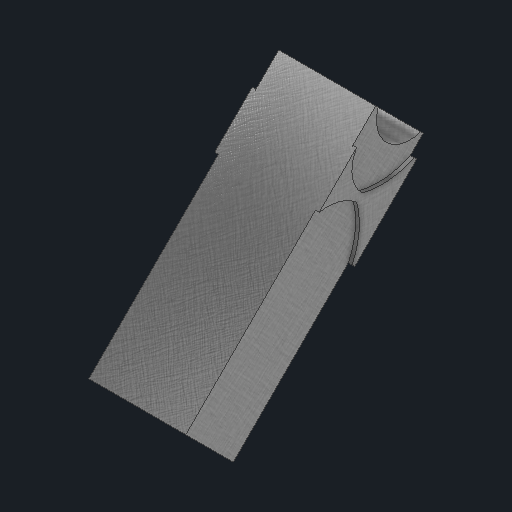
# Autodesk Inventor part: McCrea_paza_Walle
Saved by Autodesk Inventor 2022 (Build 260153000, 153)
## iProperties
Created: 2022-01-25
Part Number: McCrea_paza_Walle
Material: Generic
Document SubType Name: Modeling
Designer: Lukas
Density: 1 g/cm^3
Appearance: Honed - Dark Gray
Author: Lukas
Autodesk Inventor part; units mm, degrees
ref_plane "YZ Plane" through (0, 0, 0) normal (1, 0, 0) x (0, 1, 0)
ref_plane "XZ Plane" through (0, 0, 0) normal (0, 1, 0) x (-1, 0, 0)
ref_plane "XY Plane" through (0, 0, 0) normal (0, 0, 1) x (1, 0, 0)
sketch "Sketch1" plane through (0, 0, 0) normal (1, 0, 0) x (0, 1, 0)
  line L0 (0, 0) -> (6.364, 6.364)
  line L1 (0, 0) -> (10.533, 0) construction
  line L2 (0, 0) -> (36, 0) construction
  line L3 (-19.0919, 31.8198) -> (-25.4558, 25.4558)
  line L4 (-19.0919, 31.8198) -> (6.364, 6.364)
  line L5 (-25.4558, 25.4558) -> (0, 0)
  dimension "d0" = 9
  dimension "d1" = 45
  dimension "d2" = 36
  dimension "d15" = 9
  constraints: 12 end point, 2 horizontal, 1 parallel, 1 perpendicular, 1 point on line
  measures "d0" distance of L0.start L0.end
  measures "d1" angle of L1 L0
  measures "d2" distance of L0.start L3.end
  measures "d15" distance of L3.start L3.end
extrude "Extrusion4" add sketch "Sketch1" along normal blind 13
sketch "Sketch4" plane through (13, 0, 0) normal (1, 0, 0) x (0, 0, -1)
  line L0 (0, 0) -> (-6.364, 6.364) projected
  line L1 (-3.182, 3.182) -> (-1.7678, 1.7678)
  line L2 (-3.182, 3.182) -> (-1.7678, 4.5962)
  circle A0 centre (-1.7678, 4.5962) radius 4.5
  point P0 (-6.0324, 6.0324)
  point P1 (-0.3315, 0.3315)
  dimension "d18" = 2
  dimension "d19" = 2
  dimension "d20" = 9
  constraints: 4 end point, 1 centre point, 1 coincident, 1 midpoint, 1 perpendicular, 1 point on line
  measures "d18" distance of L1.start L1.end
  measures "d19" distance of L1.start L2.end
  measures "d20" diameter of A0
extrude "Extrusion5" cut sketch "Sketch4" against normal blind 13 contours L0 A0 picked at (-2.8444, 1.8095)
sketch "Sketch8" plane through (13, 0, 0) normal (0, -0.7071068, -0.7071068) x (-1, 0, 0)
  line L0 (0, -36) -> (0, 0) projected
  line L1 (0, -1.9255) -> (0, -2.4255)
  line L2 (0, -2.4255) -> (-0.5, -2.4255)
  line L3 (13, -36) -> (13, 0) projected
  line L4 (13, -13.6899) -> (13, -14.1899)
  line L5 (13, -14.1899) -> (13.5, -14.1899)
  line L6 (13.5, -14.1899) -> (-0.5, -14.1899)
  line L7 (-0.5, -14.1899) -> (-0.5, -2.4255)
  line L8 (-0.5, -2.4255) -> (13.5, -2.4255)
  line L9 (13.5, -2.4255) -> (13.5, -14.1899)
  dimension "d31" = 0.5
  dimension "d32" = 0.5
  dimension "d33" = 0.5
  dimension "d34" = 0.5
  constraints: 16 end point, 4 point on line, 2 horizontal, 2 parallel, 2 perpendicular
  measures "d31" distance of L1.start L1.end
  measures "d32" distance of L1.end L2.end
  measures "d33" distance of L4.start L4.end
  measures "d34" distance of L4.end L5.end
extrude "Extrusion7" add sketch "Sketch8" along normal blind 0.5
sketch "Sketch9" plane through (13, 0, 0) normal (1, 0, 0) x (0, 0, -1)
  line L0 (-1.7151, -1.7151) -> (-10.0338, -10.0338) projected
  line L1 (-5.8744, -5.8744) -> (-12.2384, 0.4895)
  line L2 (-6.364, 6.364) -> (-31.8198, -19.0919) projected
  line L3 (-9.0564, -2.6925) -> (-8.7029, -2.3389)
  line L4 (-9.0564, -2.6925) -> (-9.41, -3.046)
  line L5 (-1.7151, -1.7151) -> (0, 0) projected
  arc A0 (-8.7029, -2.3389) -> (-1.7151, -1.7151) centre (-6.0417, 7.3005) ccw
  arc A1 (-10.0338, -10.0338) -> (-9.41, -3.046) centre (-19.0494, -5.7072) ccw
  arc A2 (-9.41, -3.046) -> (-14.443, -1.7151) centre (-13.3407, -7.7285) ccw
  arc A3 (-9.41, 3.3179) -> (-8.7029, -2.3389) centre (-5.3886, 0.948) ccw
  dimension "d37" = 0.5
  dimension "d38" = 0.5
  dimension "d39" = 10
  dimension "d40" = 10
  constraints: 8 point on circle, 6 end point, 4 centre point, 3 point on line, 2 midpoint, 1 perpendicular
  measures "d37" distance of L3.start L3.end
  measures "d38" distance of L3.start L4.end
  measures "d39" radius of A0
  measures "d40" radius of A1
extrude "Extrusion8" add sketch "Sketch9" along normal blind 0.5 and the other way blind 13.5
body "Solid2"
